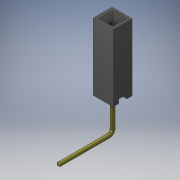
# Autodesk Inventor part: Buchsenleiste_female_90_2
Saved by Autodesk Inventor 2017 SP1 (Build 210196100, 196)
## iProperties
Part Number: Buchsenleiste_female_90_2
Material: Generisch
Document SubType Name: Modeling
Designer: Alex
Density: 1 g/cm^3
Appearance: Vorgabe
Author: Alex
Autodesk Inventor part; units mm, degrees
ref_plane "YZ Plane" through (0, 0, 0) normal (1, 0, 0) x (0, 1, 0)
ref_plane "XZ Plane" through (0, 0, 0) normal (0, 1, 0) x (-1, 0, 0)
ref_plane "XY Plane" through (0, 0, 0) normal (0, 0, 1) x (1, 0, 0)
sketch "Skizze1" plane through (0, 0, 0) normal (0, 0, 1) x (1, 0, 0)
  line L0 (0, 0) -> (2.54, 0)
  line L1 (2.54, 0) -> (2.54, -2.4)
  line L2 (2.54, -2.4) -> (0, -2.4)
  line L3 (0, -2.4) -> (0, 0)
  dimension "d0" = 2.54
  dimension "d1" = 2.4
  constraints: 8 end point, 2 parallel, 1 horizontal, 1 perpendicular
  measures "d0" distance of L1.end L2.end
  measures "d1" distance of L0.end L1.end
extrude "Extrusion1" add sketch "Skizze1" along normal blind 8.5
sketch "Skizze2" plane through (0, 0, 8.5) normal (0, 0, 1) x (-1, 0, 0)
  line L0 (-0.97, 0.9) -> (-1.57, 0.9)
  line L1 (-1.57, 0.9) -> (-1.57, 1.5)
  line L2 (-1.57, 1.5) -> (-0.97, 1.5)
  line L3 (-0.97, 1.5) -> (-0.97, 0.9)
  line L4 (0, 2.4) -> (-2.54, 2.4) projected
  line L5 (0, 2.4) -> (0, 0) projected
  dimension "d4" = 0.6
  dimension "d5" = 0.6
  dimension "d6" = 0.9
  dimension "d7" = 0.97
  constraints: 8 end point, 2 parallel, 1 horizontal, 1 perpendicular
  measures "d4" distance of L1.end L2.end
  measures "d5" distance of L0.end L1.end
  measures "d6" distance between parallel lines of L4 L2
  measures "d7" distance between parallel lines of L5 L3
extrude "Extrusion2" cut sketch "Skizze2" against normal blind 6.5
chamfer "Fase1" distance 0.6 angle 45 4 edges at (1.27, -1.5, 8.5) (0.97, -1.2, 8.5) (1.27, -0.9, 8.5) (1.57, -1.2, 8.5)
sketch "Skizze4" plane through (0, 0, 0) normal (0, 0, -1) x (-1, 0, 0)
  line L0 (-2.54, 0) -> (-2.54, -2.4) projected
  line L1 (0, -0.7) -> (-2.54, -0.7)
  line L2 (-2.54, -0.7) -> (-2.54, -1.7)
  line L3 (-2.54, -1.7) -> (0, -1.7)
  line L4 (0, -1.7) -> (0, -0.7)
  line L5 (-2.54, -2.4) -> (0, -2.4) projected
  point P0 (0, 0)
  dimension "d18" = 1
  dimension "d19" = 0.7
  constraints: 8 end point, 2 parallel, 1 horizontal, 1 perpendicular, 1 point on line
  measures "d18" distance between parallel lines of L3 L1
  measures "d19" distance between parallel lines of L5 L3
extrude "Extrusion4" cut sketch "Skizze4" against normal blind 0.5
fillet "Rundung1" radius 0.05 16 edges at (1.27, -1.7, 0.5) (1.27, -0.7, 0.5) (1.57, -1.2, 7.9) (1.27, -1.5, 7.9) (0.97, -1.2, 7.9) (1.27, -0.9, 7.9) (1.27, -2.1, 8.5) (0.67, -1.8, 8.2) (0.37, -1.2, 8.5) (1.27, -0.3, 8.5) (2.17, -1.2, 8.5) (1.87, -0.6, 8.2) (1.87, -1.8, 8.2) (0.67, -0.6, 8.2) (1.27, -1.7, 0) (1.27, -0.7, 0)
ref_plane "Arbeitsebene1" through (0, 0, 7.5) normal (0, 0, 1) x (-1, 0, 0)
split_face "Trennen1"
ref_plane "Arbeitsebene2" through (1.27, -0.05, 0) normal (-1, 0, 0) x (0, -1, 0)
sketch "Skizze3" plane through (0, 0, 0.5) normal (0, 0, -1) x (-1, 0, 0)
  line L0 (-1.57, -0.9) -> (-1.57, -1.5)
  line L1 (-0.97, -0.9) -> (-1.57, -0.9)
  line L2 (-0.97, -1.5) -> (-0.97, -0.9)
  line L3 (-1.57, -1.5) -> (-0.97, -1.5)
  circle A0 centre (-1.27, -1.2) radius 0.25
  point P0 (0, 0)
  dimension "d13" = 0.5
  dimension "d14" = 0.3
  dimension "d15" = 0.3
  constraints: 8 end point, 1 centre point
  measures "d13" diameter of A0
  measures "d14" distance from line of L2 A0.centre
  measures "d15" distance from line of L1 A0.centre
sketch "Skizze5" plane through (1.27, -0.05, 0) normal (-1, 0, 0) x (0, -1, 0)
  line L0 (1.15, 0.5) -> (1.15, -3.64)
  arc A0 (1.15, -3.64) -> (1.65, -4.14) centre (1.65, -3.64) ccw
  line L1 (1.65, -3.64) -> (1.65, -4.14) construction
  line L2 (1.65, -3.64) -> (1.15, -3.64) construction
  line L3 (1.65, -4.14) -> (8.09, -4.14)
  line L4 (1.65, -4.14) -> (8.09, -4.14) construction
  line L5 (2.35, 0) -> (2.35, 8.5) projected
  line L6 (2.35, 0) -> (1.7, 0) projected
  point P0 (2.35, 0.05)
  point P1 (2.35, 8.45)
  point P2 (2.3, 0)
  dimension "d35" = 90
  dimension "d36" = 0.5
  dimension "d38" = 5.74
  dimension "d39" = 4.14
  constraints: 10 end point, 3 horizontal, 2 point on circle, 1 centre point, 1 collinear, 1 vertical
  measures "d35" angle of L2 L1
  measures "d36" distance of L0.end L1.start
  measures "d38" distance from line of L3.end L5
  measures "d39" distance between parallel lines of L6 L3
sweep "Sweeping1" add profiles "Skizze3" path "Skizze5" path curves L0 A0 L3 contours A0
chamfer "Fase4" distance 0.15 angle 45 1 edges at (1.52, -8.14, -4.14)
